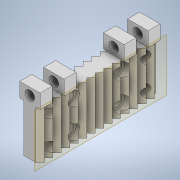
# Autodesk Inventor part: beltTensionerMid
Saved by Autodesk Inventor 2020 (Build 240168000, 168)
## iProperties
Created: 2020-01-19
Part Number: beltTensionerMid
Material: Generic
Document SubType Name: Modeling
Designer: PAB
Density: 1 g/cm^3
Appearance: Default
Author: PAB
Autodesk Inventor part; units mm, degrees
ref_plane "XZ Plane" through (0, 0, 0) normal (0, 1, 0) x (-1, 0, 0)
ref_plane "XY Plane" through (0, 0, 0) normal (0, 0, 1) x (1, 0, 0)
sketch "Sketch1" plane through (0, 0, 0) normal (0, 1, 0) x (-1, 0, 0)
  line L0 (2.5, 25) -> (-2.5, 25)
  line L1 (-2.5, 25) -> (-2.5, -25)
  line L2 (-2.5, -25) -> (2.5, -25)
  line L3 (2.5, -25) -> (2.5, 25)
  point P0 (0, 0)
  dimension "d0" = 5
  dimension "d1" = 50
  constraints: 8 end point, 2 parallel, 1 horizontal, 1 perpendicular
  measures "d0" distance of L2.end L1.end
  measures "d1" distance of L1.end L0.end
extrude "Extrusion1" add sketch "Sketch1" along normal blind 20
sketch "Sketch2" plane through (0, 20, 0) normal (0, 1, 0) x (1, 0, 0)
  line L0 (-2.5, -25) -> (2.5, -25) projected
  line L1 (2.5, -25) -> (4.2678, -23.2322)
  line L2 (2.5, -25) -> (5, -25) construction
  line L3 (4.2678, -23.2322) -> (2.5, -21.4645)
  line L4 (2.5, -25) -> (2.5, 25) projected
  line L5 (2.5, -21.4645) -> (4.2678, -19.6967)
  line L6 (4.2678, -19.6967) -> (2.5, -17.9289)
  line L7 (2.5, -17.9289) -> (4.2678, -16.1612)
  line L8 (4.2678, -16.1612) -> (2.5, -14.3934)
  line L9 (2.5, -14.3934) -> (4.2678, -12.6256)
  line L10 (4.2678, -12.6256) -> (2.5, -10.8579)
  line L11 (2.5, -10.8579) -> (4.2678, -9.0901)
  line L12 (4.2678, -9.0901) -> (2.5, -7.3223)
  line L13 (2.5, -7.3223) -> (4.2678, -5.5546)
  line L14 (4.2678, -5.5546) -> (2.5, -3.7868)
  line L15 (2.5, -3.7868) -> (4.2678, -2.019)
  line L16 (4.2678, -2.019) -> (2.5, -0.2513)
  line L17 (2.5, -0.2513) -> (4.2678, 1.5165)
  line L18 (4.2678, 1.5165) -> (2.5, 3.2843)
  line L19 (2.5, 3.2843) -> (4.2678, 5.052)
  line L20 (4.2678, 5.052) -> (2.5, 6.8198)
  line L21 (2.5, 6.8198) -> (4.2678, 8.5876)
  line L22 (4.2678, 8.5876) -> (2.5, 10.3553)
  line L23 (2.5, 10.3553) -> (4.2678, 12.1231)
  line L24 (4.2678, 12.1231) -> (2.5, 13.8909)
  line L25 (2.5, 13.8909) -> (4.2678, 15.6586)
  line L26 (4.2678, 15.6586) -> (2.5, 17.4264)
  line L27 (2.5, 17.4264) -> (4.2678, 19.1942)
  line L28 (4.2678, 19.1942) -> (2.5, 20.9619)
  line L29 (2.5, 20.9619) -> (4.2678, 22.7297)
  line L30 (4.2678, 22.7297) -> (2.5, 24.4975)
  line L31 (2.5, 24.4975) -> (2.5, -25)
  point P0 (0, 0)
  dimension "d4" = 2.5
  dimension "d5" = 45
  constraints: 60 end point, 27 perpendicular, 1 equal length, 1 horizontal, 1 vertical, 2 other
  measures "d4" distance of L0.end L1.end
  measures "d5" angle of L2 L1
extrude "Extrusion2" add sketch "Sketch2" against normal blind 20
mirror "Mirror1" about plane through (0, 0, 0) normal (1, 0, 0) of "Extrusion2"
sketch "Sketch3" plane through (0, 0, 0) normal (1, 0, 0) x (0, 1, 0)
  circle A0 centre (4, 10) radius 2
  circle A1 centre (4, -10) radius 2
  circle A2 centre (16, 10) radius 2
  circle A3 centre (16, -10) radius 2
  point P0 (0, 0)
  dimension "d8" = 4
  dimension "d9" = 4
  dimension "d10" = 4
  dimension "d11" = 4
  constraints: 4 centre point
  measures "d8" diameter of A0
  measures "d9" diameter of A1
  measures "d10" diameter of A2
  measures "d11" diameter of A3
extrude "Extrusion3" cut sketch "Sketch3" against normal mid plane 30
ref_plane "Work Plane1" through (4.4, 0, 0) normal (1, 0, 0) x (0, 1, 0)
sketch "Sketch4" plane through (4.4, 0, 0) normal (1, 0, 0) x (0, 1, 0)
  arc A0 (14.219, 9.0901) -> (17.781, 9.0901) centre (16, 10) ccw projected
  circle A1 centre (16, 10) radius 3
  arc A2 (2.219, 9.0901) -> (5.781, 9.0901) centre (4, 10) ccw projected
  circle A3 centre (4, 10) radius 3
  arc A4 (14.0318, -10.3553) -> (17.9682, -10.3553) centre (16, -10) ccw projected
  circle A5 centre (16, -10) radius 3
  arc A6 (5.416, -8.5876) -> (2.584, -8.5876) centre (4, -10) ccw projected
  circle A7 centre (4, -10) radius 3
  point P0 (0, 0)
  dimension "d15" = 6
  dimension "d16" = 6
  dimension "d17" = 6
  dimension "d18" = 6
  constraints: 4 centre point, 4 coincident
  measures "d15" diameter of A1
  measures "d16" diameter of A3
  measures "d17" diameter of A5
  measures "d18" diameter of A7
extrude "Extrusion4" cut sketch "Sketch4" against normal blind 3
mirror "Mirror2" about plane through (0, 0, 0) normal (1, 0, 0) of "Extrusion4"
sketch "Sketch5" plane through (4.4, 0, 0) normal (1, 0, 0) x (0, 1, 0)
  circle A0 centre (16, 20) radius 2
  circle A1 centre (16, -20) radius 2
  circle A2 centre (4, -20) radius 2
  circle A3 centre (4, 20) radius 2
  point P0 (0, 0)
  dimension "d21" = 4
  dimension "d22" = 4
  dimension "d23" = 4
  dimension "d24" = 4
  constraints: 4 centre point
  measures "d21" diameter of A0
  measures "d22" diameter of A1
  measures "d23" diameter of A2
  measures "d24" diameter of A3
extrude "Extrusion5" cut sketch "Sketch5" against normal blind 20
sketch "Sketch6" plane through (0, 20, 0) normal (0, 1, 0) x (1, 0, 0)
  line L0 (4.268, -25) -> (-4.268, -25)
  line L1 (-4.268, -25) -> (-4.268, -20)
  line L2 (-4.268, -20) -> (4.268, -20)
  line L3 (4.268, -20) -> (4.268, -25)
  line L4 (4.268, -15) -> (-4.268, -15)
  line L5 (-4.268, -15) -> (-4.268, -10)
  line L6 (-4.268, -10) -> (4.268, -10)
  line L7 (4.268, -10) -> (4.268, -15)
  point P0 (0, 0)
  dimension "d27" = 8.536
  dimension "d28" = 5
  dimension "d29" = 8.536
  dimension "d30" = 5
  constraints: 16 end point, 4 parallel, 2 horizontal, 2 perpendicular
  measures "d27" distance of L1.end L2.end
  measures "d28" distance of L0.end L1.end
  measures "d29" distance of L5.end L6.end
  measures "d30" distance of L4.end L5.end
extrude "Extrusion6" add sketch "Sketch6" along normal blind 6
mirror "Mirror3" about plane through (0, 0, 0) normal (0, 0, 1) of "Extrusion6"
sketch "Sketch7" plane through (2.5, 0, -25) normal (0, 0, -1) x (-1, 0, 0)
  circle A0 centre (2.5, 23) radius 2
  point P0 (2.5, 0)
  dimension "d33" = 4
  constraints: 1 centre point
  measures "d33" diameter of A0
extrude "Extrusion7" cut sketch "Sketch7" against normal blind 50
body "Solid1"
